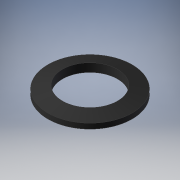
# Autodesk Inventor part: C-AC-WASHERS-M8
Saved by Autodesk Inventor 2019 (Build 230136000, 136)
## iProperties
Created: 2023-10-14
Part Number: C-AC-WASHERS-M8
Material: Generic
Catalog Web Link: www.cadenas.de
Description: C-AC-WASHERS-C-AC-WASHERS
Vendor: MISUMI
Document SubType Name: Modeling
Designer: psAdmin
Manufacturer: MISUMI
Mass: 0.0784613 g
Surface Area: 2.21215 cm^2
Volume: 0.0784613 cm^3
Density: 1 g/cm^3
Appearance: PSOLRGB-175-175-175
Category: PARTsolutions
Company: MISUMI
Title: C-AC-WASHERS-M8
Author: Cadenas PARTsolutions
Comments: C-AC-WASHERS
PSOL_IDENT_0: {$CADENAS_DATA/23d-libs/misumi/metric/29_springs/c_ac____/c_ac_____washers.prj},176 {VTYP=3D},{NB=C-
PSOL_IDENT_1: AC-WASHERS-M8},{LINA=C-AC-WASHERS-M8},{NN=C-AC-WASHERS},{DATE=28.09.2022 00:58:44},{GEOMDATE=18.03.2
PSOL_IDENT_2: 021 05:27:50},{VERSION=},{LINEID=30},{WBVAR=},{WBNUMERIC=}  {NB=C-AC-WASHERS-M8},{LINA=C-AC-WASHERS-
PSOL_IDENT_3: M8},{KT=DUMMY},{PN=C-AC-WASHERS-M8},{N=M8},{D=13.0},{DD=8.5},{TT=0.8},{H=1.3},{M=8}
NB: C-AC-WASHERS-M8
NN: C-AC-WASHERS
NT: C-AC-WASHERS
NBSYN: $PN.
LINA: C-AC-WASHERS-M8
CATALOG: Misumi
N: M8
D: 13
DD: 8.5
TT: 0.8
H: 1.3
SUPPLIER: MISUMI
ARTICLENO: C-AC-WASHERS-M8
BOMINFO: C-AC-WASHERS-M8
CREATOR: CADENAS GmbH
Autodesk Inventor part; units mm, degrees
sketch "_____1" plane through (0, 0, 0) normal (0, 0, 1) x (1, 0, 0)
  line L0 (0, -13) -> (0, 13)
  line L1 (4.25, 1.3) -> (4.25, 0)
  line L2 (4.25, 0) -> (6.5, 0)
  line L3 (6.5, 0) -> (6.5, 0.8)
  line L4 (6.5, 0.8) -> (4.25, 1.3)
  constraints: 10 end point
revolve "Revolution1" add sketch "_____1" angle 360 about axis through (0, -13, 0) along (0, -1, 0)
ref_plane "to_body1_XY" through (0, 0, 0) normal (0, 1, 0) x (1, 0, 0)
ref_plane "to_body1_YZ" through (0, 0, 0) normal (1, 0, 0) x (0, 0, -1)
ref_plane "to_body1_ZX" through (0, 0, 0) normal (0, 0, -1) x (0, 1, 0)
ref_plane "to_bolt2_XY" through (0, 0, 0) normal (0, 1, 0) x (1, 0, 0)
ref_plane "to_bolt2_YZ" through (0, 0, 0) normal (1, 0, 0) x (0, 0, -1)
ref_plane "to_bolt2_ZX" through (0, 0, 0) normal (0, 0, -1) x (0, 1, 0)
body "Solid1"
